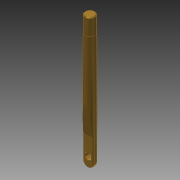
# Autodesk Inventor part: Link Arm 2
Saved by Autodesk Inventor 2013 (Build 170138000, 138)
## iProperties
Created: 2012-10-29
Part Number: Link Arm 2
Material: Generic
Document SubType Name: Modeling
Designer: uqgtayle
Density: 1 g/cm^3
Author: uqgtayle
Autodesk Inventor part; units mm, degrees
ref_plane "XZ Plane" through (0, 0, 0) normal (0, 1, 0) x (-1, 0, 0)
ref_plane "XY Plane" through (0, 0, 0) normal (0, 0, 1) x (1, 0, 0)
sketch "Sketch1" plane through (0, 0, 0) normal (0, 0, 1) x (1, 0, 0)
  circle A0 centre (0, 0) radius 1.55
  dimension "d0" = 3.1
  constraints: 1 centre point, 1 coincident
  measures "d0" diameter of A0
extrude "Extrusion1" add sketch "Sketch1" against normal blind 40
ref_plane "Work Plane1" through (2, 0, 0) normal (1, 0, 0) x (0, 1, 0)
sketch "Sketch2" plane through (2, 0, 0) normal (1, 0, 0) x (0, 1, 0)
  line L0 (-1.55, -40) -> (1.55, -40) projected
  line L1 (1.55, 0) -> (1.55, -40) projected
  line L2 (-1.55, 0) -> (-1.55, -40) projected
  line L3 (-0.6268, -40) -> (-0.6268, -31.5)
  line L4 (-0.6268, -31.5) -> (-1.55, -23)
  line L5 (0.6686, -40) -> (0.6686, -31.5)
  line L6 (0.6686, -31.5) -> (1.55, -23)
  point P0 (0, 0)
  dimension "d5" = 8.5
  dimension "d7" = 8.5
  dimension "d8" = 17
  dimension "d9" = 17
  constraints: 8 end point, 4 point on line, 2 parallel
  measures "d5" distance of L3.start L3.end
  measures "d7" distance of L5.start L5.end
  measures "d8" vertical distance of L4.end L3.start
  measures "d9" vertical distance of L6.end L5.start
extrude "Extrusion2" cut sketch "Sketch2" against normal through all
fillet "Fillet1" radius 1.5 2 edges at (1.5165, -0.3203, -40) (1.5116, 0.3428, -40)
sketch "Sketch3" plane through (-1.3984, 0.6686, -31.5) normal (0, 1, 0) x (1, 0, 0)
  point P0 (1.3984, -31.5)
  point P1 (1.3984, 5.5)
hole "Hole1" at (0, 0.6686, -37) direction (0, -1, 0) diameter 2 end through all
sketch "Sketch4" plane through (0, 0, 0) normal (0, 0, 1) x (1, 0, 0)
  circle A0 centre (0, 0) radius 1.55 projected
  circle A1 centre (0, 0) radius 1.5
  dimension "d20" = 3
  constraints: 1 centre point, 1 coincident
  measures "d20" diameter of A1
extrude "Extrusion3" cut sketch "Sketch4" against normal blind 5
chamfer "Chamfer1" distance 0.25 angle 45 1 edges at (-1.5, 0, 0)
body "Solid1"
